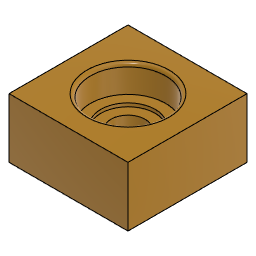
CubeBlock v2 v2 (Autodesk Fusion 360 design; units mm, degrees)
Autodesk Fusion 360 part; units mm, degrees
note: some values were not read from the file. Chosen so that the rebuilt part matches the saved one: a direction.
sketch "Sketch2" plane through (0, 0, 0) normal (0, 0, 1) x (1, 0, 0)
  line L0 (17.5, 17.5) -> (-17.5, 17.5)
  line L1 (-17.5, 17.5) -> (-17.5, -17.5)
  line L2 (-17.5, -17.5) -> (17.5, -17.5)
  line L3 (17.5, -17.5) -> (17.5, 17.5)
  line L4 (17.5, 17.5) -> (-17.5, -17.5) construction
  line L5 (-17.5, 17.5) -> (17.5, -17.5) construction
  dimension "d10" = 35
  dimension "d11" = 35
  constraint horizontal L0
  constraint perpendicular L0 L1
  constraint parallel L0 L2
  constraint parallel L1 L3
  constraint coincident L4 origin
  constraint coincident L5 origin
  measures "d10" distance of L0.end L1.end
  measures "d11" distance of L0.start L0.end
extrude "Extrude2" add sketch "Sketch2" along normal blind 17.5
sketch "Sketch3" plane through (0, 0, 17.5) normal (0, 0, 1) x (-1, 0, 0)
  line L0 (-17.5, 17.5) -> (-17.5, -17.5)
  line L1 (-17.5, -17.5) -> (17.5, -17.5)
  line L2 (17.5, -17.5) -> (17.5, 17.5)
  line L3 (17.5, 17.5) -> (-17.5, 17.5)
  circle A0 centre (0, 0) radius 11.05
  dimension "d14" = 22.1
  constraint coincident A0.centre origin
  measures "d14" diameter of A0
extrude "Extrude3" cut sketch "Sketch3" against normal blind 8 contours A0
sketch "Sketch4" plane through (0, 0, 9.5) normal (0, 0, 1) x (-1, 0, 0)
  circle A0 centre (0, 0) radius 11.05
  circle A1 centre (0, 0) radius 8
  dimension "d20" = 16
  constraint concentric A0 A1
  measures "d20" diameter of A1
extrude "Extrude4" cut sketch "Sketch4" against normal blind 1 contours A1
sketch "Sketch5" plane through (0, 0, 8.5) normal (0, 0, 1) x (-1, 0, 0)
  circle A0 centre (0, 0) radius 8
  circle A1 centre (0, 0) radius 5
  dimension "d23" = 10
  constraint concentric A0 A1
  measures "d23" diameter of A1
extrude "Extrude5" cut sketch "Sketch5" against normal through all contours A1
fillet "Fillet1" radius 1 1 edges at (10.3022, -3.9959, 17.5)
equation "TOL = 0.1 mm"
equation "BlockSize = 35 mm"
equation "d10 = BlockSize"
equation "d11 = BlockSize"
equation "d12 = BlockSize / 2"
equation "d14 = BearingOuter + TOL"
equation "d15 = -( BearingDepth + 1 mm )"
equation "BearingOuter = 22 mm"
equation "BearingInner = 8 mm"
equation "BearingWall = 2 mm"
equation "d20 = BearingOuter - BearingWall * 3"
equation "d23 = BearingInner + 2 mm"
equation "BearingDepth = 7 mm"
